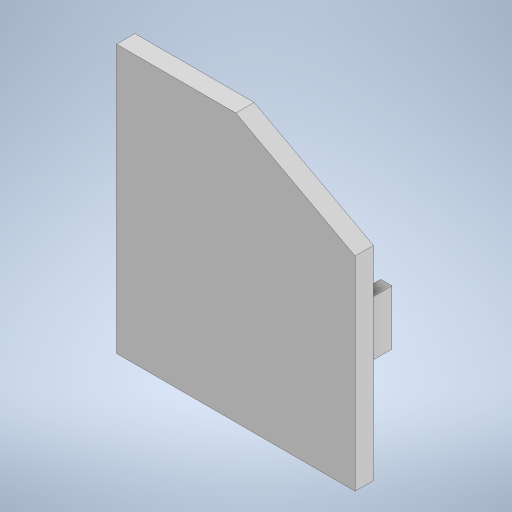
# Autodesk Inventor part: Afsluitklep
Saved by Autodesk Inventor 2024 (Build 280153000, 153)
## iProperties
Created: 2024-05-26
Part Number: Afsluitklep
Material: Generic
Document SubType Name: Modeling
Designer: 12302093
Density: 1 g/cm^3
Appearance: Default
Author: 12302093
Autodesk Inventor part; units mm, degrees
ref_plane "YZ Plane" through (0, 0, 0) normal (1, 0, 0) x (0, 1, 0)
ref_plane "XZ Plane" through (0, 0, 0) normal (0, 1, 0) x (-1, 0, 0)
ref_plane "XY Plane" through (0, 0, 0) normal (0, 0, 1) x (1, 0, 0)
sketch "Sketch1" plane through (0, 0, 0) normal (0, 0, 1) x (1, 0, 0)
  line L0 (0, 175.2) -> (0, -29.2) projected
  line L1 (-91, 0) -> (91, 0) projected
  line L2 (0, 0) -> (-65, 0)
  line L3 (-65, 0) -> (-65, 146)
  line L4 (0, 0) -> (65, 0)
  line L5 (65, 0) -> (65, 111)
  line L6 (-65, 146) -> (0, 146)
  line L7 (0, 146) -> (65, 111)
  dimension "d0" = 65
  dimension "d1" = 146
  dimension "d2" = 65
  dimension "d3" = 111
  dimension "d4" = 65
  constraints: 12 end point, 3 point on line, 1 perpendicular, 1 vertical
  measures "d0" distance of L2.start L2.end
  measures "d1" distance of L2.end L3.end
  measures "d2" distance of L2.start L4.end
  measures "d3" distance of L4.end L5.end
  measures "d4" distance of L3.end L6.end
extrude "Extrusion1" add sketch "Sketch1" along normal blind 10
sketch "Sketch2" plane through (0, 0, 0) normal (0, 0, -1) x (-1, 0, 0)
  line L0 (0, -29.2) -> (0, 175.2) projected
  line L1 (-91, 0) -> (91, 0) projected
  line L2 (65, 146) -> (65, 0) projected
  line L3 (0, 146) -> (65, 146) projected
  line L4 (-65, 111) -> (0, 146) projected
  line L5 (-65, 0) -> (-65, 111) projected
  line L6 (65, 0) -> (-65, 0) projected
  line L7 (-65, 0) -> (-55, 0)
  line L8 (-55, 0) -> (-55, 116.3846)
  line L9 (65, 0) -> (65, 10)
  line L10 (65, 10) -> (-65, 10)
  line L11 (65, 0) -> (55, 0)
  line L12 (55, 0) -> (55, 146)
  line L13 (-65, 0) -> (-65, 70)
  line L14 (-65, 70) -> (-63, 70)
  line L15 (-63, 70) -> (-63, 85)
  line L16 (-63, 85) -> (-57, 85)
  line L17 (-57, 85) -> (-57, 55)
  line L18 (-57, 55) -> (-63, 55)
  line L19 (-63, 55) -> (-63, 70)
  line L20 (65, 0) -> (65, 70)
  line L21 (65, 70) -> (63, 70)
  line L22 (63, 70) -> (63, 85)
  line L23 (63, 85) -> (57, 85)
  line L24 (57, 85) -> (57, 55)
  line L25 (57, 55) -> (63, 55)
  line L26 (63, 70) -> (63, 55)
  line L27 (0, 0) -> (0, 2)
  line L28 (0, 2) -> (-20, 2)
  line L29 (-20, 2) -> (-20, 8)
  line L30 (-20, 8) -> (20, 8)
  line L31 (20, 8) -> (20, 2)
  line L32 (20, 2) -> (0, 2)
  dimension "d7" = 10
  dimension "d8" = 10
  dimension "d9" = 10
  dimension "d10" = 70
  dimension "d11" = 2
  dimension "d12" = 15
  dimension "d13" = 6
  dimension "d14" = 30
  dimension "d15" = 70
  dimension "d16" = 2
  dimension "d17" = 15
  dimension "d18" = 6
  dimension "d19" = 30
  dimension "d20" = 2
  dimension "d21" = 20
  dimension "d22" = 6
  dimension "d23" = 40
  constraints: 52 end point, 17 point on line, 12 perpendicular, 1 collinear, 1 parallel
  measures "d7" distance of L5.start L7.end
  measures "d8" distance of L2.end L9.end
  measures "d9" distance of L2.end L11.end
  measures "d10" distance of L5.start L13.end
  measures "d11" distance of L13.end L14.end
  measures "d12" distance of L14.end L15.end
  measures "d13" distance of L15.end L16.end
  measures "d14" distance of L16.end L17.end
  measures "d15" distance of L2.end L20.end
  measures "d16" distance of L20.end L21.end
  measures "d17" distance of L21.end L22.end
  measures "d18" distance of L22.end L23.end
  measures "d19" distance of L23.end L24.end
  measures "d20" distance of L27.start L27.end
  measures "d21" distance of L27.end L28.end
  measures "d22" distance of L28.end L29.end
  measures "d23" distance of L29.end L30.end
extrude "Extrusion2" add sketch "Sketch2" along normal blind 12 contours L28 L29 L30 L0 | L0 L30 L31 L32 | L15 L16 L17 L18 L19 | L26 L25 L24 L23 L22
body "Solid1"
